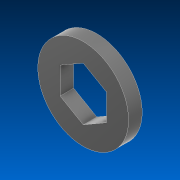
# Autodesk Inventor part: 1_10 Spacer 1_2 Hex Custom
Saved by Autodesk Inventor 2022.2 (Build 262287000, 287)
## iProperties
Created: 2022-03-21
Part Number: 1_10 Spacer 1_2 Hex Custom
Material: PET Plastic
Document SubType Name: Modeling
Designer: omard
Density: 1.541 g/cm^3
Appearance: Smooth - Black
Author: omard
Autodesk Inventor part; units mm, degrees
ref_plane "YZ Plane" through (0, 0, 0) normal (1, 0, 0) x (0, 1, 0)
ref_plane "XZ Plane" through (0, 0, 0) normal (0, 1, 0) x (-1, 0, 0)
ref_plane "XY Plane" through (0, 0, 0) normal (0, 0, 1) x (1, 0, 0)
sketch "Sketch1" plane through (0, 0, 0) normal (0, 0, 1) x (1, 0, 0)
  circle A0 centre (0, 0) radius 12.7
  line L0 (0, -7.479) -> (-6.477, -3.7395)
  line L1 (-6.477, -3.7395) -> (-6.477, 3.7395)
  line L2 (-6.477, 3.7395) -> (0, 7.479)
  line L3 (0, 7.479) -> (6.477, 3.7395)
  line L4 (6.477, 3.7395) -> (6.477, -3.7395)
  line L5 (6.477, -3.7395) -> (0, -7.479)
  dimension "d0" = 12.954
  dimension "d1" = 25.4
  constraints: 12 end point, 2 coincident, 1 centre point, 1 vertical alignment, 13 other
  measures "d0" distance between parallel lines of L1 L4
  measures "d1" diameter of A0
extrude "Extrusion1" add sketch "Sketch1" along normal blind 3.81
body "Solid1"
